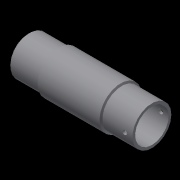
# Autodesk Inventor part: BackPair1PistonBody
Saved by Autodesk Inventor 2015 SP1 (Build 190203100, 203)
## iProperties
Created: 2014-09-27
Part Number: BackPair1PistonBody
Material: Generic
Document SubType Name: Modeling
Designer: Inventor
Mass: 9.71512 g
Surface Area: 80.2492 cm^2
Volume: 9.71512 cm^3
Density: 1 g/cm^3
Appearance: Default
Author: Inventor
Autodesk Inventor part; units mm, degrees
ref_plane "YZ Plane" through (0, 0, 0) normal (1, 0, 0) x (0, 1, 0)
ref_plane "XZ Plane" through (0, 0, 0) normal (0, 1, 0) x (-1, 0, 0)
ref_plane "XY Plane" through (0, 0, 0) normal (0, 0, 1) x (1, 0, 0)
sketch "Profile" plane through (0, 0, 0) normal (0, 0, 1) x (1, 0, 0)
  line L0 (-16.8, 0) -> (-16.8, 11)
  line L1 (-16.8, 11) -> (0, 11)
  line L2 (0, 11) -> (0.5774, 12)
  line L3 (0.5774, 12) -> (35.5774, 12)
  line L4 (35.5774, 12) -> (36.1547, 11)
  line L5 (36.1547, 11) -> (53.2, 11)
  line L6 (53.2, 11) -> (53.2, 0)
  line L7 (-16.8, 0) -> (0, 0)
  line L8 (0, 0) -> (0, 9)
  line L9 (0, 9) -> (45.2, 9)
  line L10 (45.2, 9) -> (45.2, 0)
  line L11 (45.2, 0) -> (53.2, 0)
  line L12 (-30.8, 0) -> (67.2, 0) construction
  line L13 (0, 11) -> (0, 9) construction
  dimension "BodyLength" = 70
  dimension "d1" = 11
  dimension "d3" = 120
  dimension "d4" = 120
  dimension "d5" = 35
  dimension "d6" = 16.8
  dimension "d16" = 8
  dimension "d29" = 1
  dimension "d30" = 9
  constraints: 26 end point, 6 perpendicular, 3 point on line, 2 collinear, 1 horizontal, 1 parallel, 1 vertical
  measures "BodyLength" distance between parallel lines of L6 L0
  measures "d1" distance of L0.start L0.end
  measures "d3" angle of L3 L2
  measures "d4" angle of L3 L4
  measures "d5" distance of L2.end L3.end
  measures "d6" distance of L0.end L1.end
  measures "d16" distance between parallel lines of L6 L10
  measures "d29" distance between parallel lines of L3 L5
  measures "d30" distance between parallel lines of L12 L9
revolve "ProfileRevolveFeature" add sketch "Profile" angle 360 about axis through (-10, 0, 0) along (1, 0, 0)
sketch "InsideHole" plane through (-16.8, 0, 0) normal (-1, 0, 0) x (0, 0, 1)
  circle A0 centre (0, 0) radius 9 construction
hole "InsideHoleFeature" at (-16.8, 0, 0) direction (1, 0, 0) diameter 19 end through all
chamfer "EndChamferFeature" distance 1 angle 45 1 edges at (-16.8, -11, 0)
sketch "CapMountHole" plane through (0, 0, 0) normal (0, 1, 0) x (-1, 0, 0)
  line L0 (-53.2, 11) -> (-53.2, -11) construction
  line L1 (11.4, 0) -> (-68.4, 0) construction
  circle A0 centre (-48.7, 0) radius 1.25
  point P0 (0, 0)
  dimension "d31" = 4.5
  dimension "d39" = 2.5
  constraints: 1 centre point, 1 coincident, 1 point on line
  measures "d31" distance from line of L0 point (-48.7, 0)
  measures "d39" diameter of A0
extrude "CapMountHoleFeature" cut sketch "CapMountHole" along normal through all both and the other way through all
equation "\"d5\" = 0.5 * BodyLength"
equation "\"d6\" = 0.24 * BodyLength"
